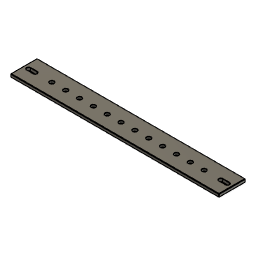
array bottom bracket (Autodesk Fusion 360 design; units mm, degrees)
Autodesk Fusion 360 part; units mm, degrees
note: some values were not read from the file. Set by a fixed rule: which sketch regions a step uses.
sketch "Sketch1" plane through (0, 0, 0) normal (0, 1, 0) x (1, 0, 0)
  line L0 (0, 0) -> (-313.2, 0)
  line L1 (-313.2, 0) -> (-313.2, -39.8)
  line L2 (-313.2, -39.8) -> (0, -39.8)
  line L3 (0, -39.8) -> (0, 0)
  line L4 (0, -19.9) -> (-313.2, -19.9) construction
  line L5 (-7.2, -17.2) -> (-17.2, -17.2)
  line L6 (-17.2, -22.6) -> (-7.2, -22.6)
  arc A0 (-17.2, -17.2) -> (-17.2, -22.6) centre (-17.2, -19.9) ccw
  arc A1 (-7.2, -22.6) -> (-7.2, -17.2) centre (-7.2, -19.9) ccw
  point P0 (-12.2, -19.9)
  point P1 (-42.2, -19.9)
  dimension "d1" = 39.8
  dimension "d11" = 313.2
  dimension "d14" = 5.4
  dimension "d15" = 5.4
  dimension "d17" = 7.2
  dimension "d18" = 10
  dimension "d19" = 10
  dimension "d20" = 5.4
  dimension "d21" = 12.2
  dimension "d30" = 25
  constraint horizontal L0
  constraint vertical L1
  constraint horizontal L2
  constraint vertical L3
  constraint coincident L0.start L3.end
  constraint midpoint L3 L4.start
  constraint midpoint L1 L4.end
  constraint coincident L4 A1.centre
  constraint coincident L4 A0.centre
  constraint horizontal L5
  constraint parallel L5 L6
  constraint coincident L4 P0
  constraint coincident L4 P1
  measures "d1" distance of L0.start L2.end
  measures "d11" distance of L0.start L0.end
  measures "d14" diameter of A1
  measures "d15" diameter of A0
  measures "d17" distance of L3 A1.centre
  measures "d18" distance of A1.centre A0.centre
  measures "d19" distance of L6.start L6.end
  measures "d20" distance of L5.end L6.start
  measures "d21" distance of L3 P0
  measures "d30" distance of A0.centre P1
extrude "Extrude1" add sketch "Sketch1" against normal blind 4.8 contours L0 L1 L2 L3 | L5 L6 A0 A1
hole "Hole1" at (-42.2, 0, 19.9) direction (0, -1, 0) diameter 3.5 end through all counterbore diameter 6 counterbore depth 3.2
chamfer "Chamfer1" distance 0.4 angle 45 2 edges at (-41.1152, 0, 17.103) (-42.8328, -4.8, 18.2684)
pattern_linear "R-Pattern1" count 12 spacing 20.8 along (-1, 0, 0) of "Hole1", "Chamfer1"
extrude "Extrude2" cut sketch "Sketch1" against normal up to surface (4.8 mm away) contours L5 L6 A0 A1
chamfer "Chamfer2" distance 0.4 angle 45 8 edges at (-12.2, 0, 17.2) (-4.5, 0, 19.9) (-12.2, 0, 22.6) (-19.9, 0, 19.9) (-4.5, -4.8, 19.9) (-12.2, -4.8, 17.2) (-19.9, -4.8, 19.9) (-12.2, -4.8, 22.6)
pattern_linear "R-Pattern2" count 2 spacing 288.8 along (-1, 0, 0) of "Extrude2", "Chamfer2"
chamfer "Chamfer3" distance 0.6 angle 45 12 edges at (0, 0, 19.9) (-156.6, 0, 0) (0, -4.8, 19.9) (0, -2.4, 0) (-156.6, -4.8, 0) (-156.6, -4.8, 39.8) (-156.6, 0, 39.8) (0, -2.4, 39.8) (-313.2, -4.8, 19.9) (-313.2, -2.4, 0) (-313.2, 0, 19.9) (-313.2, -2.4, 39.8)
equation "numHoles = 12"
equation "d11 = length"
equation "length = ( ( 7.2 + 10 ) * 2 ) * 1 mm + 50 mm + ( 20.8 * ( numHoles - 1 ) ) * 1 mm"
equation "d34 = numHoles"
equation "d40 = length - ( 7.2 mm - ( 5.4 / 2 ) * 1 mm ) - ( 15.4 mm ) - ( 7.2 mm - ( 5.4 / 2 ) * 1 mm )"
